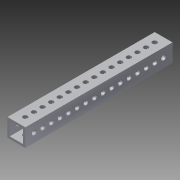
# Autodesk Inventor part: Chassis Part9 (26x28)
Saved by Autodesk Inventor 2014 SP1 (Build 180222100, 222)
## iProperties
Created: 2013-01-18
Part Number: Chassis Part9 (26x28)
Material: Aluminum 6061
Document SubType Name: Modeling
Designer: Moses
Mass: 150.857 g
Surface Area: 377.382 cm^2
Volume: 55.6669 cm^3
Density: 2.71 g/cm^3
Appearance: Aluminum - Flat
Author: Moses
Autodesk Inventor part; units mm, degrees
ref_plane "YZ Plane" through (0, 0, 0) normal (1, 0, 0) x (0, 1, 0)
ref_plane "XZ Plane" through (0, 0, 0) normal (0, 1, 0) x (-1, 0, 0)
ref_plane "XY Plane" through (0, 0, 0) normal (0, 0, 1) x (1, 0, 0)
sketch "Sketch1" plane through (0, 0, 0) normal (0, 0, 1) x (1, 0, 0)
  line L0 (0, 0) -> (25.4, 0)
  line L1 (25.4, 0) -> (25.4, 25.4)
  line L2 (25.4, 25.4) -> (0, 25.4)
  line L3 (0, 25.4) -> (0, 0)
  line L4 (3.175, 22.225) -> (22.225, 22.225)
  line L5 (22.225, 22.225) -> (22.225, 3.175)
  line L6 (22.225, 3.175) -> (3.175, 3.175)
  line L7 (3.175, 3.175) -> (3.175, 22.225)
  dimension "d0" = 25.4
  dimension "d1" = 25.4
  dimension "d2" = 3.175
  constraints: 16 end point, 4 parallel, 2 perpendicular, 1 horizontal, 3 other
  measures "d0" distance of L2.end L1.end
  measures "d1" distance of L1.end L0.end
  measures "d2" distance between parallel lines of L1 L5
extrude "Extrusion1" add sketch "Sketch1" along normal blind 209.55
sketch "Sketch2" plane through (25.4, 0, 0) normal (1, 0, 0) x (0, 0, -1)
  line L0 (0, 0) -> (0, 25.4) projected
  line L1 (-209.55, 0) -> (-209.55, 25.4) projected
  line L2 (0, 0) -> (-209.55, 0) projected
  line L3 (-209.55, 12.7) -> (-196.85, 12.7) construction
  line L4 (0, 12.7) -> (-12.7, 12.7) construction
  circle A0 centre (-196.85, 12.7) radius 3.302
  line L5 (0, 25.4) -> (-209.55, 25.4) projected
  line L6 (-196.85, 12.7) -> (-12.7, 12.7) construction
  circle A1 centre (-184.5733, 12.7) radius 3.302
  circle A2 centre (-172.2967, 12.7) radius 3.302
  circle A3 centre (-160.02, 12.7) radius 3.302
  circle A4 centre (-147.7433, 12.7) radius 3.302
  circle A5 centre (-135.4667, 12.7) radius 3.302
  circle A6 centre (-123.19, 12.7) radius 3.302
  circle A7 centre (-110.9133, 12.7) radius 3.302
  circle A8 centre (-98.6367, 12.7) radius 3.302
  circle A9 centre (-86.36, 12.7) radius 3.302
  circle A10 centre (-74.0833, 12.7) radius 3.302
  circle A11 centre (-61.8067, 12.7) radius 3.302
  circle A12 centre (-49.53, 12.7) radius 3.302
  circle A13 centre (-37.2533, 12.7) radius 3.302
  circle A14 centre (-24.9767, 12.7) radius 3.302
  circle A15 centre (-12.7, 12.7) radius 3.302
  dimension "d5" = 12.7
  dimension "d7" = 6.604
  dimension "d13" = 209.55
  dimension "d16" = 12.2767
  constraints: 16 centre point, 6 end point, 2 coincident, 2 midpoint, 2 parallel, 1 collinear, 1 horizontal, 30 other
  measures "d5" distance of L3.start L3.end
  measures "d7" diameter of A0
  measures "d13" distance of L0.end L1.end
  measures "d16" distance of L6.start A1.centre
extrude "Extrusion2" cut sketch "Sketch2" against normal through all contours A0 | A1 | A2 | A3 | A4 | A5 | A6 | A7 | A8 | A9 | A10 | A11 | A12 | A13 | A14 | A15
sketch "Sketch3" plane through (0, 0, 0) normal (0, -1, 0) x (1, 0, 0)
  line L0 (0, 0) -> (25.4, 0) projected
  line L1 (0, 209.55) -> (25.4, 209.55) projected
  line L2 (12.7, 209.55) -> (12.7, 0) construction
  circle A0 centre (12.7, 196.85) radius 3.302
  circle A1 centre (12.7, 184.5733) radius 3.302
  circle A2 centre (12.7, 172.2967) radius 3.302
  circle A3 centre (12.7, 160.02) radius 3.302
  circle A4 centre (12.7, 147.7433) radius 3.302
  circle A5 centre (12.7, 135.4667) radius 3.302
  circle A6 centre (12.7, 123.19) radius 3.302
  circle A7 centre (12.7, 110.9133) radius 3.302
  circle A8 centre (12.7, 98.6367) radius 3.302
  circle A9 centre (12.7, 86.36) radius 3.302
  circle A10 centre (12.7, 74.0833) radius 3.302
  circle A11 centre (12.7, 61.8067) radius 3.302
  circle A12 centre (12.7, 49.53) radius 3.302
  circle A13 centre (12.7, 37.2533) radius 3.302
  circle A14 centre (12.7, 24.9767) radius 3.302
  circle A15 centre (12.7, 12.7) radius 3.302
  dimension "d21" = 12.7
  dimension "d22" = 209.55
  dimension "d23" = 6.604
  dimension "d26" = 12.2767
  constraints: 16 centre point, 2 end point, 2 midpoint, 1 point on line, 1 vertical, 30 other
  measures "d21" distance from line of L1 A0.centre
  measures "d22" distance of L0.end L1.end
  measures "d23" diameter of A0
  measures "d26" distance of A0.centre A1.centre
extrude "Extrusion3" cut sketch "Sketch3" against normal blind 25.4
equation "\"d26\" = -0.133333 * d21 + 0.0666667 * d22"
body "Solid1"
